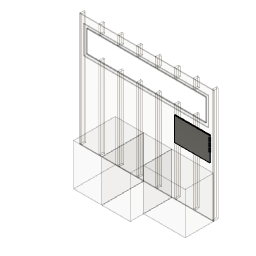
model (Autodesk Fusion 360 design; units mm, degrees)
Autodesk Fusion 360 part; units mm, degrees
note: some values were not read from the file. Chosen so that the rebuilt part matches the saved one: which bodies a step acts on. Set by a fixed rule: which sketch regions a step uses.
sketch "Sketch1" plane through (0, 0, 0) normal (0, 0, 1) x (1, 0, 0) in component "wall"
  line L0 (0, 0) -> (38.1, 0)
  line L1 (38.1, 0) -> (38.1, 88.9)
  line L2 (38.1, 88.9) -> (0, 88.9)
  line L3 (0, 88.9) -> (0, 0)
  line L4 (406.4, 88.9) -> (406.4, 0)
  line L5 (406.4, 0) -> (444.5, 0)
  line L6 (444.5, 88.9) -> (406.4, 88.9)
  line L7 (444.5, 0) -> (444.5, 88.9)
  line L8 (812.8, 88.9) -> (812.8, 0)
  line L9 (812.8, 0) -> (850.9, 0)
  line L10 (850.9, 88.9) -> (812.8, 88.9)
  line L11 (850.9, 0) -> (850.9, 88.9)
  line L12 (1219.2, 88.9) -> (1219.2, 0)
  line L13 (1219.2, 0) -> (1257.3, 0)
  line L14 (1257.3, 88.9) -> (1219.2, 88.9)
  line L15 (1257.3, 0) -> (1257.3, 88.9)
  line L16 (1625.6, 88.9) -> (1625.6, 0)
  line L17 (1625.6, 0) -> (1663.7, 0)
  line L18 (1663.7, 88.9) -> (1625.6, 88.9)
  line L19 (1663.7, 0) -> (1663.7, 88.9)
  line L20 (2032, 88.9) -> (2032, 0)
  line L21 (2032, 0) -> (2070.1, 0)
  line L22 (2070.1, 88.9) -> (2032, 88.9)
  line L23 (2070.1, 0) -> (2070.1, 88.9)
  line L24 (2438.4, 88.9) -> (2438.4, 0)
  line L25 (2438.4, 0) -> (2476.5, 0)
  line L26 (2476.5, 88.9) -> (2438.4, 88.9)
  line L27 (2476.5, 0) -> (2476.5, 88.9)
  line L28 (2844.8, 88.9) -> (2844.8, 0)
  line L29 (2844.8, 0) -> (2882.9, 0)
  line L30 (2882.9, 88.9) -> (2844.8, 88.9)
  line L31 (2882.9, 0) -> (2882.9, 88.9)
  line L32 (1986.9, -12.7) -> (2882.9, -12.7)
  line L33 (2882.9, -12.7) -> (2882.9, -620.7)
  line L34 (2882.9, -620.7) -> (1986.9, -620.7)
  line L35 (1986.9, -620.7) -> (1986.9, -12.7)
  line L36 (1378.9, -12.7) -> (1986.9, -12.7)
  line L37 (1986.9, -12.7) -> (1986.9, -908.7)
  line L38 (1986.9, -908.7) -> (1378.9, -908.7)
  line L39 (1378.9, -908.7) -> (1378.9, -12.7)
  line L40 (770.9, -12.7) -> (1378.9, -12.7)
  line L41 (1378.9, -12.7) -> (1378.9, -908.7)
  line L42 (1378.9, -908.7) -> (770.9, -908.7)
  line L43 (770.9, -908.7) -> (770.9, -12.7)
  line L44 (0, 0) -> (2882.9, 0)
  line L45 (2882.9, 0) -> (2882.9, -12.7)
  line L46 (2882.9, -12.7) -> (0, -12.7)
  line L47 (0, -12.7) -> (0, 0)
  dimension "d1" = 38.1
  dimension "d2" = 88.9
  dimension "d5" = 406.4
  dimension "d6" = 0
  dimension "d9" = 608
  dimension "d10" = 896
  dimension "d11" = 896
  dimension "d12" = 608
  dimension "d13" = 896
  dimension "d14" = 608
  dimension "d23" = 12.7
  constraint horizontal L0
  constraint vertical L1
  constraint horizontal L2
  constraint vertical L3
  constraint coincident L0.start L3.end
  constraint horizontal L32
  constraint vertical L33
  constraint horizontal L34
  constraint vertical L35
  constraint horizontal L36
  constraint vertical L37
  constraint horizontal L38
  constraint vertical L39
  constraint horizontal L40
  constraint vertical L41
  constraint horizontal L42
  constraint vertical L43
  constraint collinear L31 L33
  constraint horizontal L44
  constraint vertical L45
  constraint horizontal L46
  constraint vertical L47
  constraint collinear L31 L45
  constraint coincident L32.end L33.start
  measures "d1" distance of L1.end L2.end
  measures "d2" distance of L0.start L2.end
  measures "d9" distance of L32.end L33.end
  measures "d10" distance of L33.end L34.end
  measures "d11" distance of L32.start L37.end
  measures "d12" distance of L32.start L36.start
  measures "d13" distance of L36.start L38.end
  measures "d14" distance of L36.start L40.start
  measures "d23" distance of L29.end L32.end
extrude "Extrude1" add sketch "Sketch1" along normal blind 2438.4 contours L0 L1 L2 L3 L44 | L4 L5 L6 L7 L44 | L8 L9 L10 L11 L44 | L12 L13 L14 L15 L44 | L28 L29 L30 L31 L44 | L16 L17 L18 L19 L44 | L24 L25 L26 L27 L44 | L20 L21 L22 L23 L44 makes body 1 at (1625.6, 59.2667, 812.8) makes body 2 at (812.8, 59.2667, 812.8) makes body 3 at (2438.4, 59.2667, 812.8) makes body 4 at (1219.2, 59.2667, 812.8) makes body 5 at (2844.8, 59.2667, 812.8) makes body 6 at (0, 59.2667, 812.8) makes body 7 at (406.4, 59.2667, 812.8) makes body 8 at (2032, 59.2667, 812.8) in component "wall"
extrude "Extrude2" add sketch "Sketch1" along normal up to surface (2438.4 mm away) separate body contours L0 L5 L9 L13 L17 L21 L25 L29 L32 L36 L40 L44 L45 L46 L47 makes body 9 in component "wall"
extrude "Extrude3" add sketch "Sketch1" along normal blind 900 separate body contours L39 L40 L41 L42 L43 L46 | L32 L33 L34 L35 L37 L46 makes body 10 at (1378.9, -610.0333, 600) makes body 11 at (2285.5667, -12.7, 300) in component "wall"
extrude "Extrude4" add sketch "Sketch1" along normal up to surface (900 mm away) separate body contours L35 L36 L37 L38 L39 L41 L46 makes body 12 in component "wall"
sketch "Sketch2" plane through (0, -12.7, 0) normal (0, -1, 0) x (1, 0, 0) in component "wall"
  line L0 (2882.9, 2438.4) -> (0, 2438.4)
  line L1 (0, 2438.4) -> (0, 0)
  line L2 (0, 0) -> (2882.9, 0)
  line L3 (2882.9, 0) -> (2882.9, 2438.4)
  line L4 (1986.9, 900) -> (2882.9, 900)
  line L5 (100, 2300) -> (2782.9, 2300)
  line L6 (2782.9, 2300) -> (2782.9, 1700)
  line L7 (2782.9, 1700) -> (100, 1700)
  line L8 (100, 1700) -> (100, 2300)
  line L9 (2722.9, 1760) -> (160, 1760)
  line L10 (160, 1760) -> (160, 2240)
  line L11 (160, 2240) -> (2722.9, 2240)
  line L12 (2722.9, 2240) -> (2722.9, 1760)
  dimension "d49" = 100
  dimension "d50" = 100
  dimension "d51" = 800
  dimension "d52" = 600
  dimension "d53" = 60
  constraint horizontal L5
  constraint vertical L6
  constraint horizontal L7
  constraint vertical L8
  measures "d49" distance of L3 L6
  measures "d50" distance of L1 L8
  measures "d51" distance of L4 L7
  measures "d52" distance of L5 L7
extrude "Extrude8" cut sketch "Sketch2" against normal up to surface (101.6 mm away) contours L9 L10 L11 L12 bodies 1 4 7 3 2 8 9 makes body 18 at (2032, 59.2667, 586.6667) makes body 17 at (812.8, 59.2667, 586.6667) makes body 16 at (2476.5, 29.6333, 586.6667) makes body 15 at (406.4, 59.2667, 586.6667) makes body 14 at (1219.2, 59.2667, 586.6667) makes body 13 at (1625.6, 59.2667, 586.6667) in component "wall"
extrude "Extrude9" add sketch "Sketch2" along normal blind 12 separate body contours L5 L6 L7 L8 makes body 19 in component "wall"
sketch "Sketch1 (2)" plane through (0, -12.7, 0) normal (0, -1, 0) x (1, 0, 0) in component "panels"
  line L0 (2722.9, 2240) -> (2722.9, 1760)
  line L1 (2722.9, 1760) -> (160, 1760)
  line L2 (160, 1760) -> (160, 2240)
  line L3 (160, 2240) -> (2722.9, 2240)
  line L4 (2882.9, 2438.4) -> (0, 2438.4)
  line L5 (0, 2438.4) -> (0, 0)
  line L6 (0, 0) -> (2882.9, 0)
  line L7 (2882.9, 0) -> (2882.9, 2438.4)
  line L8 (2062.9945, 1577.924) -> (2824.9945, 1577.924)
  line L9 (2824.9945, 1577.924) -> (2824.9945, 1069.924)
  line L10 (2824.9945, 1069.924) -> (2062.9945, 1069.924)
  line L11 (2062.9945, 1069.924) -> (2062.9945, 1577.924)
  dimension "d58" = 508
  dimension "d59" = 762
  constraint horizontal L8
  constraint vertical L9
  constraint horizontal L10
  constraint vertical L11
  measures "d58" distance of L8.end L9.end
  measures "d59" distance of L8.start L8.end
extrude "Extrude1'" add sketch "Sketch1 (2)" along normal blind 18 separate body contours L8 L9 L10 L11 makes body 20 in component "panels"
sketch "Sketch2 (2)" plane through (2824.9945, 0, 0) normal (1, 0, 0) x (0, 1, 0) in component "panels"
  line L0 (-12.7, 1069.924) -> (-12.7, 1577.924)
  line L1 (-12.7, 1577.924) -> (-30.7, 1577.924)
  line L2 (-30.7, 1577.924) -> (-30.7, 1069.924)
  line L3 (-30.7, 1069.924) -> (-12.7, 1069.924)
  line L4 (-42.7, 1540.724) -> (-30.7, 1528.724)
  line L5 (-30.7, 1528.724) -> (-30.7, 1479.524)
  line L6 (-30.7, 1479.524) -> (-42.7, 1491.524)
  line L7 (-42.7, 1491.524) -> (-42.7, 1540.724)
  line L8 (-30.7, 1430.324) -> (-30.7, 1381.124)
  line L9 (-30.7, 1381.124) -> (-42.7, 1393.124)
  line L10 (-42.7, 1393.124) -> (-42.7, 1442.324)
  line L11 (-42.7, 1442.324) -> (-30.7, 1430.324)
  line L12 (-30.7, 1331.924) -> (-30.7, 1282.724)
  line L13 (-30.7, 1282.724) -> (-42.7, 1294.724)
  line L14 (-42.7, 1294.724) -> (-42.7, 1343.924)
  line L15 (-42.7, 1343.924) -> (-30.7, 1331.924)
  dimension "d68" = 45
  dimension "d69" = 12
  dimension "d72" = 49.2
  dimension "d73" = 49.2
  dimension "d76" = 0
  dimension "d77" = -98.4
  constraint parallel L4 L6
  constraint vertical L7
  constraint vertical L5
  constraint collinear L2 L5
  measures "d68" angle of L4 L7
  measures "d69" distance of L5 L7
  measures "d72" distance of L4.start L6.end
  measures "d73" distance of L1.end L4.end
component "wall" placed x (1, 0, 0) y (0, 1, 0) z (0, 0, 1) at (0, 0, 0)
component "panels" placed x (1, 0, 0) y (0, 1, 0) z (0, 0, 1) at (0, 0, 0)
equation "d5 = 16\""
equation "d7 = 8'-0\""
equation "d11 = d10"
equation "d12 = d9"
equation "d13 = d11"
equation "d14 = d12"
equation "gap = 100 mm"
equation "d58 = 20\""
equation "d59 = 30\""
equation "d69 = cleatThickness"
equation "cleatThickness = 12 mm"
equation "d72 = cleatHeight"
equation "d73 = cleatHeight"
equation "d77 = -2 * cleatHeight"
equation "cleatHeight = 51 mm - 1.8 mm"
